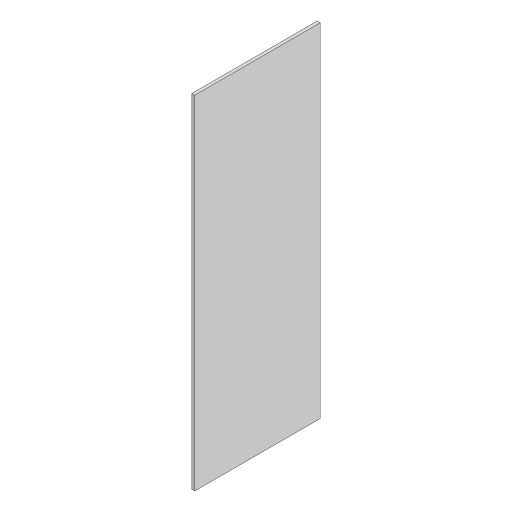
# Autodesk Inventor part: CUT PART K
Saved by Autodesk Inventor 2023.1 (Build 271208000, 208)
## iProperties
Created: 2022-11-02
Part Number: CUT PART K
Material: Generic
Document SubType Name: Modeling
Designer: GUT
Density: 1 g/cm^3
Appearance: Default
Author: GUT
Autodesk Inventor part; units mm, degrees
ref_plane "YZ Plane" through (0, 0, 0) normal (1, 0, 0) x (0, 1, 0)
ref_plane "XZ Plane" through (0, 0, 0) normal (0, 1, 0) x (-1, 0, 0)
ref_plane "XY Plane" through (0, 0, 0) normal (0, 0, 1) x (1, 0, 0)
sketch "Sketch1" plane through (0, 0, 0) normal (1, 0, 0) x (0, 1, 0)
  line L0 (-5.7461, 13.9906) -> (680.2539, 13.9906)
  line L1 (680.2539, 13.9906) -> (680.2539, -237.0094)
  line L2 (680.2539, -237.0094) -> (-5.7461, -237.0094)
  line L3 (-5.7461, -237.0094) -> (-5.7461, 13.9906)
  point P0 (0, 0)
  dimension "b" = 686
  dimension "d1" = 251
  constraints: 8 end point, 2 parallel, 1 horizontal, 1 perpendicular
  measures "b" distance of L1.end L2.end
  measures "d1" distance of L0.end L1.end
extrude "Extrusion1" add sketch "Sketch1" along normal blind 6
body "Solid1"
